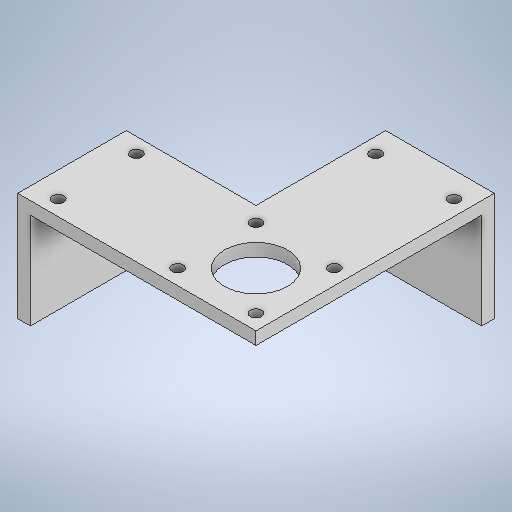
# Autodesk Inventor part: motor_holder
Saved by Autodesk Inventor 2025 (Build 290162010, 162A)
## iProperties
Created: 2025-01-16
Part Number: motor_holder
Material: Generic
Document SubType Name: Modeling
Designer: aduwa
Density: 1 g/cm^3
Appearance: Default
Author: aduwa
Autodesk Inventor part; units mm, degrees
ref_plane "YZ Plane" through (0, 0, 0) normal (1, 0, 0) x (0, 1, 0)
ref_plane "XZ Plane" through (0, 0, 0) normal (0, 1, 0) x (-1, 0, 0)
ref_plane "XY Plane" through (0, 0, 0) normal (0, 0, 1) x (1, 0, 0)
sketch "Sketch1" plane through (0, 0, 0) normal (0, 1, 0) x (1, 0, 0)
  circle A0 centre (0, 0) radius 2.25
  circle A1 centre (31, 0) radius 2.25
  circle A2 centre (0, 31) radius 2.25
  circle A3 centre (31, 31) radius 2.25
  circle A4 centre (15.5, 15.5) radius 12.5
  line L0 (-6, 37) -> (37, 37)
  line L1 (37, 37) -> (37, -6)
  line L2 (37, -6) -> (-6, -6)
  line L3 (-6, -6) -> (-6, 37)
  line L4 (-6, 37) -> (37, -6) construction
  line L5 (37, 37) -> (-6, -6) construction
  line L6 (-6, -6) -> (37, -6)
  circle A5 centre (0, 78.34) radius 2.25
  circle A6 centre (31, 78.34) radius 2.25
  line L7 (-6, 37) -> (37, 37)
  line L8 (37, 37) -> (37, 88.34)
  line L9 (37, 88.34) -> (-6, 88.34)
  line L10 (-6, 88.34) -> (-6, 37)
  line L11 (15.5, 15.5) -> (22.827, 15.5)
  line L12 (-6, 83.34) -> (37, 83.34)
  circle A7 centre (-47.34, 0) radius 2.25
  line L13 (-52.34, -6) -> (-52.34, 37)
  line L14 (-57.34, -6) -> (-6, -6)
  line L15 (-57.34, 37) -> (-57.34, -6)
  circle A8 centre (-47.34, 31) radius 2.25
  line L16 (-6, 37) -> (-57.34, 37)
  point P0 (-6, -6)
  point P1 (37, 37)
  dimension "d3" = 4.5
  dimension "d5" = 31
  dimension "d6" = 25
  dimension "d8" = 43
  dimension "d23" = 4.5
  dimension "d24" = 31
  dimension "d25" = 31
  dimension "d26" = 62.84
  dimension "d27" = 6
  dimension "d28" = 10
  dimension "d35" = 5
  dimension "d39" = 90
  constraints: 34 end point, 9 centre point, 5 horizontal, 5 point on line, 4 equal radius, 4 parallel, 3 vertical alignment, 2 horizontal alignment, 2 midpoint, 2 perpendicular, 15 other
  measures "d3" diameter of A0
  measures "d5" distance of A0.centre A2.centre
  measures "d6" diameter of A4
  measures "d8" distance of L0.end L1.end
  measures "d23" diameter of A5
  measures "d24" distance of A6.centre A5.centre
  measures "d25" distance of A1.centre A0.centre
  measures "d26" vertical distance of L11.start A6.centre
  measures "d27" distance from line of L0 A2.centre
  measures "d28" distance from line of L9 A5.centre
  measures "d35" distance between parallel lines of L9 L12
extrude "Extrusion4" add sketch "Sketch1" along normal blind 5
extrude "Extrusion5" add sketch "Sketch1" against normal blind 38 contours L10 L9 L8 L12 | L13 L14 L15 L16
body "Solid2"
